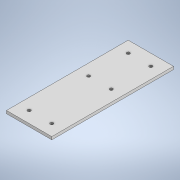
# Autodesk Inventor part: Flat Bar KY
Saved by Autodesk Inventor 2020 (Build 240168000, 168)
## iProperties
Created: 2020-01-29
Part Number: Flat Bar KY
Material: Generic
Document SubType Name: Modeling
Designer: aidan
Density: 1 g/cm^3
Appearance: Default
Author: aidan
Autodesk Inventor part; units mm, degrees
ref_plane "YZ Plane" through (0, 0, 0) normal (1, 0, 0) x (0, 1, 0)
ref_plane "XZ Plane" through (0, 0, 0) normal (0, 1, 0) x (-1, 0, 0)
ref_plane "XY Plane" through (0, 0, 0) normal (0, 0, 1) x (1, 0, 0)
sketch "Sketch1" plane through (0, 0, 0) normal (0, 0, 1) x (1, 0, 0)
  line L0 (-48.7274, 2.102) -> (2.0726, 2.102)
  line L1 (2.0726, 2.102) -> (2.0726, -1.073)
  line L2 (2.0726, -1.073) -> (-48.7274, -1.073)
  line L3 (-48.7274, -1.073) -> (-48.7274, 2.102)
  point P0 (0, 0)
  dimension "d0" = 3.175
  dimension "d1" = 50.8
  constraints: 8 end point, 2 parallel, 1 horizontal, 1 perpendicular
  measures "d0" distance of L0.end L1.end
  measures "d1" distance of L0.start L0.end
extrude "Extrusion1" add sketch "Sketch1" along normal blind 136.5504
sketch "Sketch2" plane through (-48.7274, 2.102, 0) normal (0, 1, 0) x (1, 0, 0)
  circle A0 centre (12.7, -12.7) radius 1.7653
  circle A1 centre (38.1, -12.7) radius 1.7653
  circle A2 centre (12.7, -123.8504) radius 1.7653
  circle A3 centre (38.1, -123.8504) radius 1.7653
  line L0 (12.7, -123.8504) -> (38.1, -123.8504) construction
  line L1 (38.1, -123.8504) -> (38.1, -12.7) construction
  line L2 (38.1, -12.7) -> (12.7, -12.7) construction
  line L3 (12.7, -12.7) -> (12.7, -123.8504) construction
  line L4 (50.8, 0) -> (0, 0) projected
  line L5 (50.8, 0) -> (50.8, -136.5504) projected
  point P0 (48.7274, 0)
  dimension "d5" = 3.5306
  dimension "d6" = 111.1504
  dimension "d7" = 12.7
  dimension "d8" = 25.4
  dimension "d9" = 12.7
  constraints: 8 end point, 4 centre point, 3 equal radius, 2 coincident, 2 parallel, 1 horizontal, 1 perpendicular
  measures "d5" diameter of A3
  measures "d6" distance of L0.end L1.end
  measures "d7" distance from line of L4 L1.end
  measures "d8" distance of L1.end L2.end
  measures "d9" distance between parallel lines of L5 L1
extrude "Extrusion2" cut sketch "Sketch2" against normal through all
sketch "Sketch3" plane through (-48.7274, 2.102, 0) normal (0, 1, 0) x (1, 0, 0)
  circle A0 centre (12.7, -57.15) radius 1.7272
  circle A1 centre (38.1, -57.15) radius 1.7272
  line L0 (12.7, -57.15) -> (38.1, -57.15) construction
  line L1 (0, 0) -> (0, -136.5504) projected
  circle A2 centre (12.7, -12.7) radius 1.7653 projected
  point P0 (48.7274, 0)
  point P1 (25.4, -57.15)
  dimension "d12" = 3.4544
  dimension "d13" = 25.4
  dimension "d14" = 12.7
  dimension "d15" = 44.45
  constraints: 2 centre point, 2 end point, 1 equal radius, 1 horizontal, 1 midpoint
  measures "d12" diameter of A1
  measures "d13" distance of L0.start L0.end
  measures "d14" distance from line of L1 L0.start
  measures "d15" distance of A2.centre L0.start
extrude "Extrusion3" cut sketch "Sketch3" against normal through all contours A0 | A1
equation "\"d3\" = d2"
equation "\"d2\" = 136.5504"
body "Solid1"
